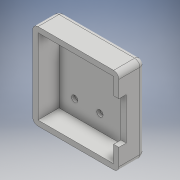
# Autodesk Inventor part: camera dcefend
Saved by Autodesk Inventor 2017 (Build 210142000, 142)
## iProperties
Part Number: camera dcefend
Material: Типовые
Document SubType Name: Modeling
Designer: TRENER
Density: 1 g/cm^3
Appearance: По умолчанию
Author: TRENER
Autodesk Inventor part; units mm, degrees
ref_plane "YZ Plane" through (0, 0, 0) normal (1, 0, 0) x (0, 1, 0)
ref_plane "XZ Plane" through (0, 0, 0) normal (0, 1, 0) x (-1, 0, 0)
ref_plane "XY Plane" through (0, 0, 0) normal (0, 0, 1) x (1, 0, 0)
sketch "Эскиз1" plane through (0, 0, 0) normal (0, 1, 0) x (-1, 0, 0)
  line L0 (0, 0) -> (36, 0)
  line L1 (36, 0) -> (36, -36)
  line L2 (36, -36) -> (0, -36)
  line L3 (0, -36) -> (0, 0)
  line L4 (0, -8) -> (-2.5, -8)
  line L5 (-2.5, -8) -> (-2.5, -28)
  line L6 (-2.5, -28) -> (0, -28)
  line L7 (0, -28) -> (0, -8)
  line L8 (-2.5, -38.5) -> (38.5, -38.5)
  line L9 (38.5, -38.5) -> (38.5, 2.5)
  line L10 (38.5, 2.5) -> (-2.5, 2.5)
  line L11 (-2.5, 2.5) -> (-2.5, -38.5)
  dimension "d0" = 36
  dimension "d1" = 36
  dimension "d2" = 2.5
  dimension "d3" = 20
  dimension "d4" = 8
  dimension "d5" = 2.5
  dimension "d6" = 2.5
  dimension "d7" = 2.5
  dimension "d8" = 2.5
  constraints: 24 end point, 6 parallel, 3 horizontal, 3 perpendicular
  measures "d0" distance of L1.end L2.end
  measures "d1" distance of L2.end L0.start
  measures "d2" distance of L6.end L5.end
  measures "d3" distance of L5.end L4.end
  measures "d4" distance between parallel lines of L2 L6
  measures "d5" distance between parallel lines of L3 L11
  measures "d6" distance between parallel lines of L2 L8
  measures "d7" distance between parallel lines of L9 L1
  measures "d8" distance between parallel lines of L10 L0
extrude "Выдавливание1" add sketch "Эскиз1" along normal blind 10 contours L3 L4 L11 L10 L9 L8 L6 L2 L1 L0
sketch "Эскиз2" plane through (0, 0, -28) normal (0, 0, 1) x (1, 0, 0)
  line L0 (0, 0) -> (0, 10) projected
  line L1 (2.5, 10) -> (2.5, 0) projected
  line L2 (0, 10) -> (2.5, 10)
  line L3 (2.5, 10) -> (2.5, 3.5)
  line L4 (2.5, 3.5) -> (0, 3.5)
  line L5 (0, 3.5) -> (0, 10)
  dimension "d11" = 6.5
  constraints: 8 end point, 2 parallel, 1 horizontal, 1 perpendicular, 1 point on line
  measures "d11" distance of L2.end L3.end
extrude "Выдавливание2" add sketch "Эскиз2" along normal blind 20
sketch "Эскиз3" plane through (0, 10, 0) normal (0, 1, 0) x (1, 0, 0)
  line L0 (2.5, -2.5) -> (2.5, 8) projected
  line L1 (2.5, 38.5) -> (-38.5, 38.5) projected
  line L2 (2.5, -2.5) -> (-38.5, -2.5)
  line L3 (-38.5, -2.5) -> (-38.5, 38.5)
  line L4 (-38.5, 38.5) -> (2.5, 38.5)
  line L5 (2.5, 38.5) -> (2.5, -2.5)
  point P0 (0, 0)
  constraints: 8 end point, 2 parallel, 1 horizontal, 1 perpendicular
extrude "Выдавливание3" add sketch "Эскиз3" along normal blind 2.5
fillet "Сопряжение1" radius 2.5 8 edges at (-38.5, 12.5, -18) (-18, 12.5, -38.5) (-38.5, 6.25, -38.5) (2.5, 6.25, -38.5) (2.5, 12.5, -18) (2.5, 6.25, 2.5) (-18, 12.5, 2.5) (-38.5, 6.25, 2.5)
sketch "Эскиз4" plane through (0, 10, 0) normal (0, -1, 0) x (1, 0, 0)
  line L0 (-36, -36) -> (-36, 0) projected
  line L1 (-36, 0) -> (0, 0) projected
  line L2 (-36, -36) -> (0, -36)
  line L3 (0, -36) -> (0, 0)
  line L4 (0, 0) -> (-36, 0)
  line L5 (-36, 0) -> (-36, -36)
  line L6 (0, -36) -> (-36, -36) projected
  line L7 (-36, -36) -> (-9, -36)
  line L8 (-9, -36) -> (-9, 0)
  line L9 (-9, 0) -> (-36, 0)
  line L10 (-36, 0) -> (-36, -36)
  line L11 (-28.5, -28.5) -> (-16.5, -28.5)
  line L12 (-16.5, -28.5) -> (-16.5, -7.5)
  line L13 (-16.5, -7.5) -> (-28.5, -7.5)
  line L14 (-28.5, -7.5) -> (-28.5, -28.5)
  circle A0 centre (-28.5, -28.5) radius 1.5
  circle A1 centre (-28.5, -7.5) radius 1.5
  circle A2 centre (-16.5, -7.5) radius 1.5
  circle A3 centre (-16.5, -28.5) radius 1.5
  dimension "d17" = 27
  dimension "d18" = 21
  dimension "d19" = 12
  dimension "d20" = 3
  dimension "d21" = 3
  dimension "d22" = 7.5
  dimension "d23" = 7.5
  dimension "d24" = 7.5
  dimension "d25" = 7.5
  dimension "d26" = 3
  dimension "d27" = 3
  constraints: 24 end point, 6 parallel, 4 centre point, 4 coincident, 3 horizontal, 3 perpendicular, 1 point on line
  measures "d17" distance of L9.end L8.end
  measures "d18" distance of L13.end L11.start
  measures "d19" distance of L12.end L13.end
  measures "d20" diameter of A0
  measures "d21" diameter of A1
  measures "d22" distance between parallel lines of L1 L13
  measures "d23" distance between parallel lines of L7 L11
  measures "d24" distance between parallel lines of L0 L14
  measures "d25" distance between parallel lines of L12 L8
  measures "d26" diameter of A2
  measures "d27" diameter of A3
extrude "Выдавливание4" cut sketch "Эскиз4" against normal blind 4 contours L14 A0 L11 | L11 A0 L14 | A3 L12 L11 | L11 L12 A3 | A1 L13 L14 | L14 L13 A1 | A2 L13 L12 | L12 L13 A2
sketch "Эскиз5" plane through (0, 12.5, 0) normal (0, 1, 0) x (1, 0, 0)
  line L0 (-28.5, 7.5) -> (-16.5, 7.5)
  line L1 (-16.5, 7.5) -> (-16.5, 28.5)
  line L2 (-16.5, 28.5) -> (-28.5, 28.5)
  line L3 (-28.5, 28.5) -> (-28.5, 7.5)
  line L4 (-36, 36) -> (0, 36) projected
  line L5 (-36, 0) -> (-36, 36) projected
  circle A0 centre (-28.5, 7.5) radius 3.06
  line L6 (-28.5, 4.44) -> (-28.5, 10.56)
  line L7 (-31.15, 5.97) -> (-31.15, 9.03)
  line L8 (-31.15, 9.03) -> (-28.5, 10.56)
  line L9 (-31.15, 5.97) -> (-28.5, 4.44)
  line L10 (-28.5, 4.44) -> (-25.85, 5.97)
  line L11 (-25.85, 5.97) -> (-25.85, 9.03)
  line L12 (-25.85, 9.03) -> (-28.5, 10.56)
  circle A1 centre (-16.5, 7.5) radius 3.06
  line L13 (-16.5, 4.44) -> (-16.5, 10.56)
  line L14 (-19.15, 5.97) -> (-19.15, 9.03)
  line L15 (-19.15, 9.03) -> (-16.5, 10.56)
  line L16 (-19.15, 5.97) -> (-16.5, 4.44)
  line L17 (-16.5, 4.44) -> (-13.85, 5.97)
  line L18 (-13.85, 5.97) -> (-13.85, 9.03)
  line L19 (-13.85, 9.03) -> (-16.5, 10.56)
  circle A2 centre (-28.5, 28.5) radius 3.06
  line L20 (-28.5, 25.44) -> (-28.5, 31.56)
  line L21 (-31.15, 26.97) -> (-31.15, 30.03)
  line L22 (-31.15, 30.03) -> (-28.5, 31.56)
  line L23 (-31.15, 26.97) -> (-28.5, 25.44)
  line L24 (-28.5, 25.44) -> (-25.85, 26.97)
  line L25 (-25.85, 26.97) -> (-25.85, 30.03)
  line L26 (-25.85, 30.03) -> (-28.5, 31.56)
  circle A3 centre (-16.5, 28.5) radius 3.06
  line L27 (-16.5, 25.44) -> (-16.5, 31.56)
  line L28 (-19.15, 26.97) -> (-19.15, 30.03)
  line L29 (-19.15, 30.03) -> (-16.5, 31.56)
  line L30 (-19.15, 26.97) -> (-16.5, 25.44)
  line L31 (-16.5, 25.44) -> (-13.85, 26.97)
  line L32 (-13.85, 26.97) -> (-13.85, 30.03)
  line L33 (-13.85, 30.03) -> (-16.5, 31.56)
  line L34 (0, 0) -> (-36, 0) projected
  circle A4 centre (-28.5, 7.5) radius 3.75
  circle A5 centre (-28.5, 28.5) radius 3.75
  circle A6 centre (-16.5, 7.5) radius 1.5 projected
  circle A7 centre (-16.5, 7.5) radius 3.75
  circle A8 centre (-16.5, 28.5) radius 1.5 projected
  circle A9 centre (-16.5, 28.5) radius 3.75
  dimension "d30" = 12
  dimension "d31" = 7.5
  dimension "d32" = 7.5
  dimension "d33" = 21
  dimension "d34" = 5.3
  dimension "d35" = 6.1199
  dimension "d36" = 5.3
  dimension "d37" = 5.3
  dimension "d38" = 5.3
  dimension "d39" = 30
  dimension "d40" = 7.5
  dimension "d41" = 7.5
  dimension "d42" = 7.5
  dimension "d43" = 7.5
  constraints: 64 end point, 24 point on circle, 18 parallel, 11 coincident, 8 centre point, 8 equal length, 1 horizontal, 1 perpendicular, 1 point on line
  measures "d30" distance of L1.end L2.end
  measures "d31" distance between parallel lines of L4 L2
  measures "d32" distance between parallel lines of L5 L3
  measures "d33" distance of L2.end L0.start
  measures "d34" distance between parallel lines of L24 L22
  measures "d35" diameter of A2
  measures "d36" distance between parallel lines of L31 L29
  measures "d37" distance between parallel lines of L16 L19
  measures "d38" distance between parallel lines of L9 L12
  measures "d39" angle of L34 L10
  measures "d40" diameter of A4
  measures "d41" diameter of A5
  measures "d42" diameter of A7
  measures "d43" diameter of A9
extrude "Выдавливание5" add sketch "Эскиз5" along normal blind 1 contours A0 L3 A4 L0 | A0 L11 L0 | L0 L11 A0 | L0 A4 L3 A0 | L12 A0 | A0 L10 | A7 L1 A1 L0 | L0 A1 L1 A7 | L8 A0 | A0 L9 | A1 L14 L0 | L0 L14 A1 | A5 L2 A2 L3 | L3 A2 L2 A5 | L7 A0 | A1 L15 | L16 A1 | A1 L19 | A9 L2 A3 L1 | L1 A3 L2 A9 | L24 A2 | A2 L23 | L17 A1 | A1 L18 | L31 A3 | A3 L30 | A2 L21 | L25 L2 A2 | L2 L25 A2 | A3 L2 L28 | L32 A3 | A3 L28 L2 | L22 A2 | A2 L26 | L33 A3 | A3 L29
sketch "Эскиз6" plane through (0, 12.5, 0) normal (0, 1, 0) x (1, 0, 0)
  line L0 (-28.5, 31.56) -> (-25.85, 30.03) projected
  line L1 (-28.5, 31.56) -> (-31.15, 30.03)
  line L2 (-31.15, 30.03) -> (-31.15, 26.97) projected
  line L3 (-31.15, 30.03) -> (-31.15, 26.97)
  line L4 (-31.15, 26.97) -> (-28.5, 25.44) projected
  line L5 (-31.15, 26.97) -> (-28.5, 25.44)
  line L6 (-25.85, 30.03) -> (-25.85, 26.97) projected
  line L7 (-28.5, 25.44) -> (-25.85, 26.97)
  line L8 (-25.85, 26.97) -> (-25.85, 30.03)
  line L9 (-25.85, 30.03) -> (-19.15, 30.03)
  line L10 (-16.5, 31.56) -> (-19.15, 30.03) projected
  line L11 (-19.15, 30.03) -> (-16.5, 31.56)
  line L12 (-16.5, 31.56) -> (-13.85, 30.03) projected
  line L13 (-16.5, 31.56) -> (-13.85, 30.03)
  line L14 (-13.85, 30.03) -> (-13.85, 26.97)
  line L15 (-13.85, 26.97) -> (-16.5, 25.44) projected
  line L16 (-13.85, 26.97) -> (-16.5, 25.44)
  line L17 (-16.5, 25.44) -> (-19.15, 26.97)
  line L18 (-19.15, 30.03) -> (-19.15, 26.97) projected
  line L19 (-19.15, 26.97) -> (-19.15, 30.03)
  line L20 (-16.5, 10.56) -> (-19.15, 9.03) projected
  line L21 (-19.15, 30.03) -> (-16.5, 10.56)
  line L22 (-13.85, 9.03) -> (-16.5, 10.56) projected
  line L23 (-16.5, 10.56) -> (-13.85, 9.03)
  line L24 (-13.85, 5.97) -> (-13.85, 9.03) projected
  line L25 (-13.85, 9.03) -> (-13.85, 5.97)
  line L26 (-19.15, 5.97) -> (-16.5, 4.44) projected
  line L27 (-13.85, 5.97) -> (-16.5, 4.44)
  line L28 (-16.5, 4.44) -> (-19.15, 5.97)
  line L29 (-19.15, 9.03) -> (-19.15, 5.97) projected
  line L30 (-19.15, 5.97) -> (-19.15, 9.03)
  line L31 (-19.15, 9.03) -> (-16.5, 10.56)
  line L32 (-25.85, 5.97) -> (-25.85, 9.03) projected
  line L33 (-25.85, 9.03) -> (-28.5, 10.56)
  line L34 (-28.5, 10.56) -> (-31.15, 9.03)
  line L35 (-28.5, 10.56) -> (-31.15, 9.03) projected
  line L36 (-31.15, 9.03) -> (-31.15, 5.97)
  line L37 (-31.15, 5.97) -> (-28.5, 4.44)
  line L38 (-28.5, 4.44) -> (-25.85, 5.97)
  line L39 (-25.85, 5.97) -> (-25.85, 9.03)
  point P0 (0, 0)
  constraints: 50 end point, 19 equal length, 2 perpendicular, 2 point on line
extrude "Выдавливание6" cut sketch "Эскиз6" against normal blind 1
fillet "Сопряжение2" radius 1 8 edges at (-32.25, 12.5, -28.5) (-20.25, 12.5, -7.5) (-32.25, 12.5, -7.5) (-20.25, 12.5, -28.5) (-32.25, 13.5, -28.5) (-32.25, 13.5, -7.5) (-20.25, 13.5, -7.5) (-20.25, 13.5, -28.5)
